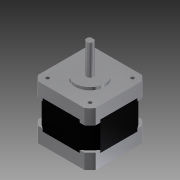
# Autodesk Inventor part: stepper
Saved by Autodesk Inventor 2013 (Build 170138000, 138)
## iProperties
Created: 2013-07-22
Part Number: stepper
Material: Generic
Document SubType Name: Modeling
Designer: employee
Density: 1 g/cm^3
Mass: 67.7183 g
Surface Area: 104.643 cm^2
Volume: 67.7183 cm^3
Author: employee
Autodesk Inventor part; units mm, degrees
ref_plane "YZ Plane" through (0, 0, 0) normal (1, 0, 0) x (0, 1, 0)
ref_plane "XZ Plane" through (0, 0, 0) normal (0, 1, 0) x (-1, 0, 0)
ref_plane "XY Plane" through (0, 0, 0) normal (0, 0, 1) x (1, 0, 0)
sketch "Sketch1" plane through (0, 0, 0) normal (0, 0, 1) x (1, 0, 0)
  line L0 (-21, 21) -> (21, 21) construction
  line L1 (21, 21) -> (21, -21) construction
  line L2 (21, -21) -> (-21, -21) construction
  line L3 (-21, -21) -> (-21, 21) construction
  line L4 (-21, 16.9706) -> (-21, -16.9706)
  line L5 (-16.9706, -21) -> (16.9706, -21)
  line L6 (21, -16.9706) -> (21, 16.9706)
  line L7 (16.9706, 21) -> (-16.9706, 21)
  arc A0 (-16.9706, 21) -> (-21, 16.9706) centre (0, 0) ccw
  arc A1 (-21, -16.9706) -> (-16.9706, -21) centre (0, 0) ccw
  arc A2 (16.9706, -21) -> (21, -16.9706) centre (0, 0) ccw
  arc A3 (21, 16.9706) -> (16.9706, 21) centre (0, 0) ccw
  dimension "d0" = 42
  dimension "d3" = 27
  constraints: 16 end point, 8 point on circle, 8 point on line, 4 centre point, 3 coincident, 3 concentric, 1 vertical, 9 other
  measures "d0" distance of L0.start L0.end
  measures "d3" radius of A2
extrude "Extrusion1" add sketch "Sketch1" along normal blind 11
sketch "Sketch2" plane through (0, 0, 11) normal (0, 0, 1) x (1, 0, 0)
  line L0 (-21, 16.9706) -> (-21, -16.9706) projected
  arc A0 (-21, -16.9706) -> (-16.9706, -21) centre (0, 0) ccw projected
  line L1 (-16.9706, -21) -> (16.9706, -21) projected
  arc A1 (16.9706, -21) -> (21, -16.9706) centre (0, 0) ccw projected
  line L2 (21, -16.9706) -> (21, 16.9706) projected
  arc A2 (21, 16.9706) -> (16.9706, 21) centre (0, 0) ccw projected
  line L3 (16.9706, 21) -> (-16.9706, 21) projected
  arc A3 (-16.9706, 21) -> (-21, 16.9706) centre (0, 0) ccw projected
  line L4 (-16.9741, 21.01) -> (16.9741, 21.01)
  arc A4 (21.01, 16.9741) -> (16.9741, 21.01) centre (0, 0) ccw
  line L5 (21.01, 16.9741) -> (21.01, -16.9741)
  arc A5 (16.9741, -21.01) -> (21.01, -16.9741) centre (0, 0) ccw
  line L6 (16.9741, -21.01) -> (-16.9741, -21.01)
  arc A6 (-21.01, -16.9741) -> (-16.9741, -21.01) centre (0, 0) ccw
  line L7 (-21.01, -16.9741) -> (-21.01, 16.9741)
  arc A7 (-16.9741, 21.01) -> (-21.01, 16.9741) centre (0, 0) ccw
  arc A8 (-13.5492, 21.01) -> (-21.01, 13.5492) centre (0, 0) ccw
  arc A9 (-21.01, -13.5492) -> (-13.5492, -21.01) centre (0, 0) ccw
  arc A10 (13.5492, -21.01) -> (21.01, -13.5492) centre (0, 0) ccw
  arc A11 (21.01, 13.5492) -> (13.5492, 21.01) centre (0, 0) ccw
  dimension "d6" = 25
  dimension "d8" = 0.01
  constraints: 16 point on circle, 8 centre point, 8 end point, 8 point on line, 3 concentric, 1 coincident, 7 other
  measures "d6" radius of A10
  measures "d8" distance between parallel lines of L0 L7
extrude "Extrusion2" add sketch "Sketch2" along normal blind 19.116 and the other way blind 2 contours A8 L3 A11 L2 A10 L1 A9 L0 | L0 A9 L7 A8 | A8 L4 A11 L3 | L1 A10 L6 A9 | A11 L5 A10 L2
sketch "Sketch3" plane through (0, 0, 30.116) normal (0, 0, 1) x (1, 0, 0)
  line L0 (-21, 16.9706) -> (-21, -16.9706) projected
  arc A0 (-16.9706, 21) -> (-21, 16.9706) centre (0, 0) ccw projected
  line L1 (16.9706, 21) -> (-16.9706, 21) projected
  arc A1 (21, 16.9706) -> (16.9706, 21) centre (0, 0) ccw projected
  line L2 (21, -16.9706) -> (21, 16.9706) projected
  arc A2 (16.9706, -21) -> (21, -16.9706) centre (0, 0) ccw projected
  line L3 (-16.9706, -21) -> (16.9706, -21) projected
  arc A3 (-21, -16.9706) -> (-16.9706, -21) centre (0, 0) ccw projected
extrude "Extrusion3" add sketch "Sketch3" along normal blind 9 and the other way blind 2
sketch "Sketch4" plane through (0, 0, 39.116) normal (0, 0, 1) x (1, 0, 0)
  arc A0 (-16.9706, 21) -> (-21, 16.9706) centre (0, 0) ccw projected
  circle A1 centre (0, 0) radius 11
  dimension "d17" = 22
  constraints: 1 centre point, 1 coincident
  measures "d17" diameter of A1
extrude "Extrusion4" add sketch "Sketch4" along normal blind 2
sketch "Sketch5" plane through (0, 0, 41.116) normal (0, 0, 1) x (1, 0, 0)
  circle A0 centre (0, 0) radius 11 projected
  circle A1 centre (0, 0) radius 2.5
  dimension "d21" = 5
  constraints: 1 centre point, 1 coincident
  measures "d21" diameter of A1
extrude "Extrusion5" add sketch "Sketch5" along normal blind 22 contours A1
sketch "Sketch6" plane through (0, 0, 63.116) normal (0, 0, 1) x (1, 0, 0)
  circle A0 centre (0, 0) radius 2.5 projected
  line L0 (-1.5, 2) -> (1.5, 2)
  dimension "d25" = 2
  constraints: 2 end point, 2 point on circle, 1 horizontal
  measures "d25" distance from line of L0 A0.centre
extrude "Extrusion6" cut sketch "Sketch6" against normal blind 15 contours L0 A0 picked at (-0.3466, 2.0912)
sketch "Sketch7" plane through (0, 0, 39.116) normal (0, 0, 1) x (1, 0, 0)
  arc A0 (-16.9706, 21) -> (-21, 16.9706) centre (0, 0) ccw projected
  line L0 (-15.5, 15.5) -> (15.5, 15.5)
  line L1 (15.5, 15.5) -> (15.5, -15.5)
  line L2 (15.5, -15.5) -> (-15.5, -15.5)
  line L3 (-15.5, -15.5) -> (-15.5, 15.5)
  dimension "d28" = 31
  constraints: 8 end point, 1 coincident, 1 horizontal, 9 other
  measures "d28" distance of L0.start L0.end
hole "Hole1" at (15.5, 15.5, 39.116) at (15.5, -15.5, 39.116) at (-15.5, -15.5, 39.116) at (-15.5, 15.5, 39.116) direction (0, 0, -1) diameter 2.459 depth 10 tip angle 118 thread size "M3x0.5" class "6H" standard "ISO Metric profile"
body "Solid1"
